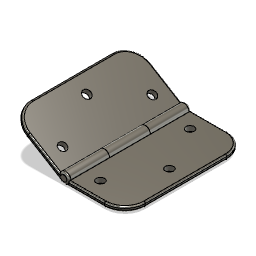
Metal_Frame_Design v2 (Autodesk Fusion 360 archive; units mm, degrees)
design "Hinge"
Autodesk Fusion 360 part; units mm, degrees
sketch "Sketch1" plane through (0, 0, 0) normal (0, 0, 1) x (1, 0, 0)
  line L0 (-9.525, 8.89) -> (25.4, 8.89)
  line L1 (25.4, 8.89) -> (25.4, 5.715)
  line L2 (25.4, 5.715) -> (-12.7, 5.715)
  arc A0 (-9.525, 8.89) -> (-12.7, 5.715) centre (-12.7, 8.89) ccw
  dimension "d2" = 38.1
  dimension "d3" = 3.175
  constraint horizontal L0
  constraint perpendicular L0 L1
  constraint perpendicular L1 L2
  constraint tangent L2 A0
  measures "d2" distance of L0.end A0.centre
  measures "d3" distance of L0.end L1.end
extrude "Extrude1" add sketch "Sketch1" along normal blind 76.2 makes body 1
sketch "Sketch2" plane through (0, 0, 76.2) normal (0, 0, 1) x (1, 0, 0)
  line L0 (25.4, 8.89) -> (-9.525, 8.89)
  arc A0 (-9.525, 8.89) -> (-12.7, 5.715) centre (-12.7, 8.89) ccw
  line L1 (-12.7, 5.715) -> (25.4, 5.715)
  line L2 (25.4, 5.715) -> (25.4, 8.89)
  circle A1 centre (-12.7, 8.89) radius 3.175
  constraint concentric A0 A1
  constraint coincident A0.end A1
extrude "Extrude2" cut sketch "Sketch2" against normal blind 25.4 contours A0 A1 bodies 1
sketch "Sketch3" plane through (0, 0, 0) normal (0, 0, -1) x (-1, 0, 0)
  line L0 (9.525, 8.89) -> (-25.4, 8.89)
  line L1 (-25.4, 8.89) -> (-25.4, 5.715)
  line L2 (-25.4, 5.715) -> (12.7, 5.715)
  arc A0 (12.7, 5.715) -> (9.525, 8.89) centre (12.7, 8.89) ccw
  circle A1 centre (12.7, 8.89) radius 3.175
  constraint concentric A0 A1
  constraint coincident L2.end A1
extrude "Extrude3" cut sketch "Sketch3" against normal blind 25.4 contours A0 A1 bodies 1
sketch "Sketch4" plane through (0, 8.89, 0) normal (0, 1, 0) x (-1, 0, 0)
  line L0 (-25.4, 0) -> (9.525, 0)
  line L1 (9.525, 0) -> (9.525, 25.4)
  line L2 (9.525, 25.4) -> (9.525, 50.8)
  line L3 (9.525, 50.8) -> (9.525, 76.2)
  line L4 (9.525, 76.2) -> (-25.4, 76.2)
  line L5 (-25.4, 76.2) -> (-25.4, 0)
  circle A0 centre (0, 10.16) radius 2.54
  circle A1 centre (-15.0622, 38.1) radius 2.54
  line L6 (-25.4, 38.1) -> (0, 38.1) construction
  circle A2 centre (0, 66.04) radius 2.54
  dimension "d10" = 5.08
  constraint midpoint L5 L6.start
  constraint perpendicular L5 L6
  constraint symmetric A0 L6 A2
  measures "d10" diameter of A1
extrude "Extrude4" cut sketch "Sketch4" against normal blind 25.4 contours A0 | A1 | A2 bodies 1
mirror "Mirror1" about plane through (0, 0, 0) normal (0, 0, 1) of bodies 1 makes body 2
copy_body "Body->Comp1" bodies 1 removing the originals makes body 3 in component "Hinge1"
copy_body "Body->Comp2" bodies 2 removing the originals makes body 4 in component "Hinge2"
extrude "Extrude1'" add 1 faces at (-12.911, 8.6786, -50.8) along direction (0, 0, -1) blind 25.4 on bodies 4 bodies 4 in component "Hinge2"
extrude "Extrude2'" add 1 faces at (-11.7284, 8.8121, -25.4) along direction (0, 0, 1) blind 25.4 on bodies 4 bodies 4 in component "Hinge2"
ref_plane "WorkPlane1" through (-11.3927, 32.9739, -63.2552) normal (0, 0, -1) x (1, 0, 0)
sketch "Sketch5" plane through (-11.3927, 32.9739, -63.2552) normal (0, 0, -1) x (1, 0, 0)
  line L0 (-14.2875, 0) -> (20.6375, 0)
  line L1 (20.6375, 0) -> (20.6375, 3.175)
  line L2 (20.6375, 3.175) -> (-17.4625, 3.175)
  arc A0 (-17.4625, 3.175) -> (-14.2875, 0) centre (-17.4625, 0) ccw
  circle A1 centre (-17.4625, 0) radius 3.175
  constraint concentric A0 A1
  constraint coincident L2.end A1
extrude "Extrude3'" cut sketch "Sketch5" against normal blind 25.4 contours A0 A1 sketch seen with x (1, 0, 0) y (0, 1, 0) z (0, 0, 1) at (16.1552, -24.0839, 12.4552) bodies 4 in component "Hinge2"
move_body "Move1" bodies 4 to x (-1, 0, 0) y (0, 1, 0) z (0, 0, -1) at (29.2088, 0, -24.4332) in component "Hinge2"
fillet "Fillet1" radius 0.889 3 edges at (7.9375, 8.89, 0) (25.4, 8.89, 38.1) (7.9375, 8.89, 76.2) on bodies 3 in component "Hinge1"
fillet "Fillet1'" radius 0.889 3 edges at (21.2713, 8.89, -24.4332) (3.8088, 8.89, 13.6668) (21.2713, 8.89, 51.7668) on bodies 4 in component "Hinge2"
fillet "Fillet2" radius 12.7 4 edges at (25.1396, 8.6296, 0.2604) (25.4, 6.858, 0) (25.4, 6.858, 76.2) (25.1396, 8.6296, 75.9396) on bodies 3 in component "Hinge1"
fillet "Fillet2'" radius 12.7 4 edges at (4.0691, 8.6296, -24.1728) (3.8088, 6.858, -24.4332) (3.8088, 6.858, 51.7668) (4.0691, 8.6296, 51.5064) on bodies 4 in component "Hinge2"
fillet "Fillet3" radius 1.27 5 edges at (0, 5.715, 0) (21.6803, 5.715, 3.7197) (25.4, 5.715, 38.1) (21.6803, 5.715, 72.4803) (0, 5.715, 76.2) on bodies 3 in component "Hinge1"
fillet "Fillet3'" radius 1.27 7 edges at (43.8138, 11.43, 51.7668) (29.2088, 5.715, 51.7668) (7.5285, 5.715, 48.0471) (3.8088, 5.715, 13.6668) (7.5285, 5.715, -20.7135) (29.2088, 5.715, -24.4332) (43.8138, 11.43, -24.4332) on bodies 4 in component "Hinge2"
component "Hinge1" placed x (1, 0, 0) y (0, 1, 0) z (0, 0, 1) at (0, 0, 0)
component "Hinge2" placed x (1, 0, 0) y (0, 1, 0) z (0, 0, 1) at (-54.6088, 0, 24.4332)
equation "d3 = ( 1 / 8 ) * 1 in"
named bodies: "Hinge1", "Hinge2"
